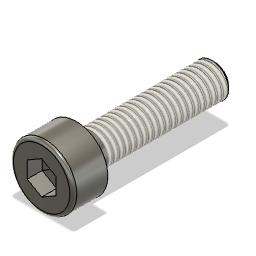
Motor_Mount v4 (Autodesk Fusion 360 archive; units mm, degrees)
design "Hexagon Socket Head Cap Screw ISO 4762 - M3 x 12 Steel 4.6 Plain"
description: Hexagon Socket Head Cap Screw ISO 4762 - M3 x 12
Autodesk Fusion 360 part; units mm, degrees
sketch "Sketch1" plane through (0, 0, 0) normal (0, 1, 0) x (1, 0, 0)
  line L0 (-1.5, 0) -> (-1.5, 12)
  line L1 (-1.5, 12) -> (0, 12)
  line L2 (0, 12) -> (0, -3)
  line L3 (-1.5, 0) -> (-2.75, 0)
  line L4 (-2.75, 0) -> (-2.75, -3)
  line L5 (-2.75, -3) -> (0, -3)
  dimension "d9" = 3
  dimension "d66" = 5.5
  dimension "d68" = 12
  dimension "d79" = 3
  constraint perpendicular L0 L1
  constraint collinear origin L1.end L2.end
  constraint perpendicular L0 L3
  constraint coincident origin L3
  constraint vertical L0
  constraint vertical L2
  constraint parallel L2 L4
  constraint coincident L2 L5.end
  constraint perpendicular L2 L5
  measures "d68" distance of origin L1.end
  measures "d79" distance of L3.end L4.end
revolve "Revolve1" add sketch "Sketch1" angle 360 about axis through (0, 0, -12) along (0, 0, 1)
ref_plane "WorkPlane1" through (0, 0, 3) normal (0, 0, 1) x (1, 0, 0)
sketch "Sketch6" plane through (0, 0, 3) normal (0, 0, 1) x (1, 0, 0)
  line L0 (-1.25, 0) -> (1.25, 0) construction
  line L1 (0, 0) -> (-1.25, 0.7217)
  line L2 (-1.25, -0.7217) -> (-1.25, 0.7217)
  line L3 (-1.25, -0.7217) -> (0, 0)
  dimension "d72" = 2.5
  dimension "d104" = 150
  constraint horizontal L0
  constraint midpoint L1.start L0
  constraint coincident L1.start L3.end
  constraint perpendicular L0 L2
  constraint midpoint L0.start L2
  constraint coincident L1.end L2.end
  measures "d72" distance of L0.start L0.end
  measures "d104" angle of L0 L1
extrude "Extrude1" cut sketch "Sketch6" against normal blind 1.3
pattern_circular "C-Pattern1" count 6 over 360 about axis through (0, 0, 1.75) along (0, 0, 1) of "Extrude1"
extrude "Extrude2" cut 1 faces at (0, -0.4811, 1.7) along direction (0, 0, -1) blind 1.3 draft -85
fillet "Fillet4" radius 0.3 1 edges at (-2.5639, 0.9944, 3)
thread "Thread2" "ISO Metric profile 3.0 M3x0.5 6g" major diameter 2.927 minor diameter 2.3555 pitch 0.5 angle 60 resizes the face on face at (-1.4925, 0.1494, -8) from (0, 0, -1.25) to (0, 0, -12)
sketch "Sketch7" plane through (0, 0, 0) normal (0, 1, 0) x (1, 0, 0)
  line L0 (-1.53, 12) -> (-1.53, 11.7)
  line L1 (-1.53, 11.7) -> (-1.23, 12)
  line L2 (0, 12) -> (0, -3)
  line L3 (-1.53, 12) -> (0, 12)
  dimension "d99" = 1.53
  dimension "d101" = 45
  dimension "d103" = 0.3
  constraint coincident L2.start L3.end
  constraint perpendicular L2 L3
  constraint coincident L1.end L3
  constraint perpendicular L0 L3
  measures "d99" distance of origin L0
  measures "d101" angle of L0 L1
  measures "d103" vertical distance of L0.end L1.end
revolve "Revolve3" cut sketch "Sketch7" angle 360 about axis through (0, 0, 1.75) along (0, 0, 1)
equation "d9 = adsk_nomdia"
equation "adsk_nomlen = 12.00 mm"
equation "adsk_headh = 3.00 mm"
equation "adsk_headdia = 5.50 mm"
equation "adsk_nomdia = 3.00 mm"
equation "adsk_philwidth = 2.50 mm"
equation "d31 = -adsk_phildepth"
equation "adsk_phildepth = 1.30 mm"
equation "d66 = adsk_headdia"
equation "d68 = adsk_nomlen"
equation "d71 = adsk_headh"
equation "d72 = adsk_philwidth"
equation "d76 = -adsk_phildepth"
equation "d79 = adsk_headh"
equation "adsk_thrlen = 10.75 mm"
equation "d84 = adsk_thrlen"
equation "d86 = adsk_nomdia * 0.1"
equation "d99 = adsk_nomdia * 0.51"
equation "adsk_startang = 45.00 deg"
equation "d101 = adsk_startang"
equation "adsk_pitch1 = 0.50 mm"
equation "d103 = adsk_startlen"
equation "adsk_startlen = 0.30 mm"

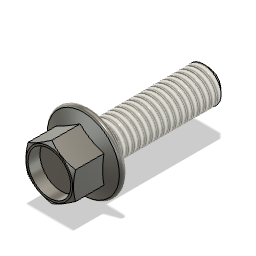
design "Indented Hex Flange Head Machine Screw ANSI B18.6.7M - M6x1 x 20 Steel Grade 2 Plain"
description: Indented Hex Flange Head Machine Screw ANSI B18.6.7M - M6x1 x 20
Autodesk Fusion 360 part; units mm, degrees
sketch "Sketch1" plane through (0, 0, 0) normal (0, 1, 0) x (1, 0, 0)
  line L0 (-3, 0) -> (-3, 20)
  line L1 (-3, 20) -> (0, 20)
  line L2 (0, 20) -> (0, -4.7)
  line L3 (-3, 0) -> (-4.62, 0)
  line L4 (-4.62, 0) -> (-4.62, -6.2959)
  line L5 (-3.92, -6.7) -> (-3.6, -6.7)
  line L6 (-3.92, -6.7) -> (-4.62, -6.2959)
  line L7 (-3.6, -6.7) -> (-3.6, -4.7)
  line L8 (-3.6, -4.7) -> (0, -4.7)
  dimension "d9" = 6
  dimension "d68" = 20
  dimension "d111" = 6.7
  dimension "d113" = 30
  dimension "d114" = 9.24
  dimension "d115" = 7.84
  dimension "d158" = 7.2
  dimension "d159" = 2
  constraint perpendicular L0 L1
  constraint perpendicular L0 L3
  constraint coincident origin L3
  constraint vertical L0
  constraint vertical L2
  constraint parallel L2 L4
  constraint coincident L2 L8.end
  constraint perpendicular L2 L5
  constraint coincident L3.end L4.start
  constraint perpendicular L5 L7
  constraint perpendicular L2 L8
  constraint coincident L2.end L8.end
  constraint coincident origin L2
  measures "d68" distance of origin L1.end
  measures "d111" distance of L3 L5
  measures "d113" angle of L5 L6
  measures "d159" distance of L5.end L7.end
revolve "Revolve1" add sketch "Sketch1" angle 360 about axis through (0, 0, -20) along (0, 0, 1)
sketch "Sketch8" plane through (0, 0, 0) normal (0, 0, 1) x (1, 0, 0)
  line L0 (0, 0) -> (-4, 0) construction
  line L1 (-4, -2.3118) -> (-4, 2.3118)
  circle A0 centre (0, 0) radius 4.62
  dimension "d110" = 4
  constraint horizontal L0
  constraint perpendicular L0 L1
  constraint coincident L0.end L1
  constraint coincident L0.start A0.centre
  constraint coincident L1.end A0
  constraint coincident L1.start A0
  measures "d110" distance of L0.start L1
extrude "Extrude5" cut sketch "Sketch8" along normal blind 6.7 contours L1 A0 picked at (-4.1, -0.5631)
pattern_circular "C-Pattern2" count 6 over 360 about axis through (0, 0, 1.75) along (0, 0, 1) of "Extrude5"
sketch "Sketch12" plane through (0, 0, 0) normal (0, 1, 0) x (1, 0, 0)
  line L0 (3.8, 0) -> (5.8845, 0)
  line L1 (6.0608, -1) -> (3.8, -1.8229)
  line L2 (3.8, -1.8229) -> (3.8, 0)
  arc A0 (6.0608, -1) -> (5.8845, 0) centre (5.8845, -0.5155) ccw
  line L3 (0, -1.75) -> (0, -22.5)
  line L4 (4.62, 0) -> (4.62, -1.5244) construction
  line L5 (0, 0) -> (4, 0)
  line L6 (6.4, 0) -> (6.4, -1.8229) construction
  line L7 (3.8, -1.8229) -> (6.4, -1.8229) construction
  dimension "d122" = 7.6
  dimension "d126" = 9.24
  dimension "d138" = 1
  dimension "d142" = 6.4
  dimension "d163" = 20
  constraint horizontal L0
  constraint perpendicular L0 L2
  constraint tangent L0 A0
  constraint tangent L1 A0
  constraint horizontal L5.start L0.start
  constraint coincident L1 L4.end
  constraint perpendicular L0 L4
  constraint coincident L0 L4.start
  constraint vertical L6
  constraint tangent A0 L6
  constraint coincident L0 L6.start
  constraint perpendicular L6 L7
  constraint coincident L6.end L7.end
  measures "d138" vertical distance of L0.end L1.start
  measures "d142" distance of L5.start L6
  measures "d163" angle of L0 L1
revolve "Revolve3" add sketch "Sketch12" angle 360 about axis through (0, 0, 1.75) along (0, 0, 1)
thread "Thread2" "ISO Metric profile 6.0 M6x1 6g" major diameter 5.884 minor diameter 4.7435 pitch 1 angle 60 resizes the face on face at (-2.9851, 0.2987, -6.6667) from (0, 0, -2.3) to (0, 0, -20)
fillet "Fillet4" radius 0.2 1 edges at (2.7429, -1.0639, 0)
sketch "Sketch5" plane through (0, 0, 0) normal (0, 1, 0) x (1, 0, 0)
  line L0 (-3.06, 19.125) -> (-2.125, 20)
  line L1 (0, -1.75) -> (0, -22.5)
  line L2 (0, 20) -> (0, -4.7)
  line L3 (0, 20) -> (-3.06, 20)
  line L4 (-3.06, 20) -> (-3.06, 19.125)
  dimension "d153" = 2.125
  dimension "d156" = 3.06
  dimension "d157" = 0.875
  constraint coincident L2.start L3.start
  constraint perpendicular L2 L3
  constraint coincident L0.end L3
  constraint perpendicular L3 L4
  measures "d153" distance of L0.end L1
  measures "d156" horizontal distance of origin L3.end
  measures "d157" distance of L0.start L3.end
revolve "Revolve2" cut sketch "Sketch5" angle 360 about axis through (0, 0, -20) along (0, 0, 1)
equation "d9 = adsk_nomdia"
equation "adsk_nomlen = 20.00 mm"
equation "adsk_headh = 6.70 mm"
equation "adsk_nomdia = 6.00 mm"
equation "d68 = adsk_nomlen"
equation "d89 = adsk_headh"
equation "adsk_waflat = 8.00 mm"
equation "d110 = adsk_waflat / 2"
equation "d111 = adsk_headh"
equation "d113 = adsk_chamang2"
equation "d114 = adsk_wacor"
equation "d115 = adsk_topdia"
equation "d122 = adsk_waflat * 0.95"
equation "d126 = adsk_waflat * 1.155"
equation "adsk_headdia = 12.80 mm"
equation "adsk_flngheig = 1.00 mm"
equation "adsk_thrlen = 17.70 mm"
equation "d133 = adsk_nomdia / 30"
equation "d138 = adsk_flngheig"
equation "d142 = adsk_headdia / 2"
equation "d144 = adsk_thrlen"
equation "adsk_endpointdia = 4.25 mm"
equation "d153 = adsk_endpointdia / 2"
equation "adsk_startlen = 0.875 mm"
equation "d156 = adsk_nomdia * 0.51"
equation "d157 = adsk_startlen"
equation "d158 = adsk_indentdia"
equation "d159 = adsk_indentdepth"
equation "adsk_wacor = 9.24 mm"
equation "adsk_topdia = adsk_waflat * 0.98"
equation "adsk_chamang2 = 30.00 deg"
equation "d163 = adsk_flngang"
equation "adsk_flngang = 20.00 deg"
equation "adsk_indentdia = 7.20 mm"
equation "adsk_indentdepth = 2.00 mm"

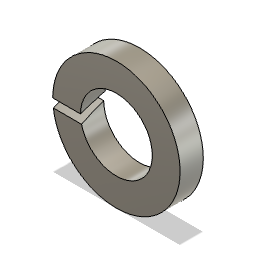
design "Spring Washer BS 4464 - M3 - Type A Steel 100 HV Plain"
description: Spring Washer BS 4464 - M3 - Type A
Autodesk Fusion 360 part; units mm, degrees
sketch "Sketch1" plane through (0, 0, 0) normal (0, 0, 1) x (1, 0, 0)
  circle A0 centre (0, 0) radius 2.75
  circle A1 centre (0, 0) radius 1.55
  dimension "d4" = 5.5
  dimension "d5" = 3.1
  constraint coincident A0.centre A1.centre
  measures "d4" diameter of A0
  measures "d5" diameter of A1
extrude "Extrude1" add sketch "Sketch1" along normal blind 1
ref_plane "WorkPlane1" through (12.125, 0, 0) normal (0, -0.34202, 0.939693) x (1, 0, 0)
ref_plane "WorkPlane2" through (12.125, -0.171, 0.4698) normal (0, -0.34202, 0.939693) x (1, 0, 0)
sketch "Sketch2" plane through (12.125, -0.171, 0.4698) normal (0, -0.34202, 0.939693) x (1, 0, 0)
  ellipse E0 centre (-12.125, 0.342) end of major axis (-9.375, 0.342) minor radius 2.5842
  ellipse E1 centre (-12.125, 0) end of major axis (-9.375, 0) minor radius 2.5842
  line L0 (-12.125, 0.342) -> (-12.125, 0)
  line L1 (-12.125, 0.342) -> (-14.985, 0.342)
  line L2 (-12.125, 0) -> (-14.985, 0)
  line L3 (-14.985, 0) -> (-14.985, 0.342)
  dimension "d15" = 2.86
  constraint coincident E0.centre L0.start
  constraint coincident E1.centre L0.end
  constraint perpendicular L0 L1
  constraint perpendicular L0 L2
  constraint vertical L3
  measures "d15" distance of L0 L3
extrude "Extrude2" cut sketch "Sketch2" along normal through all and the other way through all contours E0 E1 L1 | E0 E1 L1 L2 L3 | E0 E1 L0 L1 L2 | E0 E1 L2 picked at (-14.8608, 0.3278) picked at (-13.0336, 0.114) picked at (-14.8608, 0.0142)
equation "adsk_woutdia = 5.50 mm"
equation "adsk_windia = 3.10 mm"
equation "adsk_wthick = 1.00 mm"
equation "d4 = adsk_woutdia"
equation "d5 = adsk_windia"
equation "d6 = adsk_wthick"
equation "d13 = adsk_wthick / 2"
equation "d15 = adsk_woutdia * 0.52"
equation "d34 = adsk_wthick"
